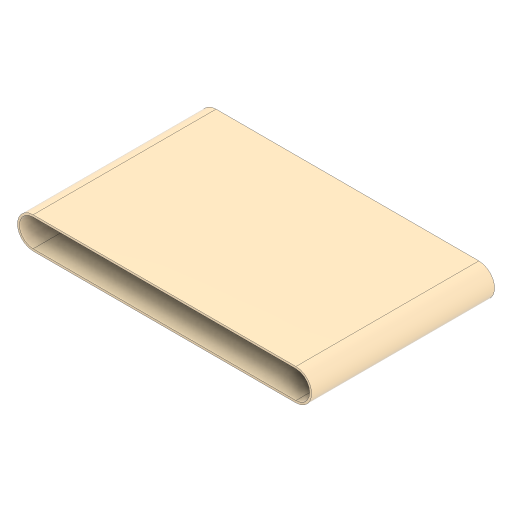
# Autodesk Inventor part: bult
Saved by Autodesk Inventor 2024 (Build 280153000, 153)
## iProperties
Created: 2023-06-14
Part Number: bult
Material: Generic
Document SubType Name: Modeling
Designer: rajen
Density: 1 g/cm^3
Appearance: Default
Author: rajen
Autodesk Inventor part; units mm, degrees
ref_plane "YZ Plane" through (0, 0, 0) normal (1, 0, 0) x (0, 1, 0)
ref_plane "XZ Plane" through (0, 0, 0) normal (0, 1, 0) x (-1, 0, 0)
ref_plane "XY Plane" through (0, 0, 0) normal (0, 0, 1) x (1, 0, 0)
sketch "Sketch1" plane through (0, 0, 0) normal (0, 0, 1) x (1, 0, 0)
  arc A0 (0, 34.29) -> (0, -34.29) centre (0, 0) ccw
  arc A1 (0, 39.37) -> (0, -39.37) centre (0, 0) ccw
  line L0 (0, 0) -> (656.8948, 0)
  arc A2 (656.8948, -34.29) -> (656.8948, 34.29) centre (656.8948, 0) ccw
  arc A3 (656.8948, -39.37) -> (656.8948, 39.37) centre (656.8948, 0) ccw
  line L1 (0, 39.37) -> (656.8948, 39.37)
  line L2 (656.8948, 34.29) -> (0, 34.29)
  line L3 (0, -34.29) -> (656.8948, -34.29)
  line L4 (656.8948, -39.37) -> (0, -39.37)
  dimension "d0" = 68.58
  dimension "d1" = 78.74
  dimension "d2" = 656.8948
  dimension "d3" = 68.58
  dimension "d4" = 78.74
  constraints: 10 end point, 8 point on circle, 6 tangent, 4 centre point, 4 coincident, 1 horizontal
  measures "d0" diameter of A0
  measures "d1" diameter of A1
  measures "d2" distance of L0.start L0.end
  measures "d3" diameter of A2
  measures "d4" diameter of A3
extrude "Extrusion1" add sketch "Sketch1" along normal blind 457.2
body "Solid1"
